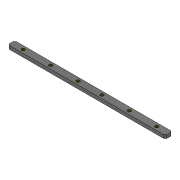
# Autodesk Inventor part: TL20240701-10100CV-003
Saved by Autodesk Inventor 2022.5 (Build 265521000, 521)
## iProperties
Category: PROFILE ASSY
Company: 현대 트랜시스
Created: 2024-04-28
Part Number: TL20240701-10100CV-003
Project: TL20240701
Checked By: 김형민
Engr Approved By: 김시현
User Status: 4 x48
Material: SS400
Description: 0
Document SubType Name: Modeling
Mfg Approved By: 호상태
Designer: 도종수
Stock Number: 003
Density: 7.85 g/cm^3
Appearance: Plating Zinc White
Folder: .\
VDS_Category: 엔지니어링
Detail Description: Processed products
Title: NUT PLATE
Subject: SW차종 시트조립라인
Author: 도종수
Revision Number: A
Autodesk Inventor part; units mm, degrees
ref_plane "YZ Plane" through (0, 0, 0) normal (1, 0, 0) x (0, 1, 0)
ref_plane "XZ Plane" through (0, 0, 0) normal (0, 1, 0) x (-1, 0, 0)
ref_plane "XY Plane" through (0, 0, 0) normal (0, 0, 1) x (1, 0, 0)
sketch "스케치52" plane through (0, 0, 0) normal (0, 0, 1) x (1, 0, 0)
  line L0 (-115, -5) -> (115, -5)
  line L1 (115, -5) -> (115, 5)
  line L2 (115, 5) -> (-115, 5)
  line L3 (-115, 5) -> (-115, -5)
  line L4 (-115, -5) -> (115, 5) construction
  line L5 (115, -5) -> (-115, 5) construction
  point P0 (0, 0)
  dimension "d480" = 230
  dimension "d481" = 10
  constraints: 12 end point, 2 midpoint, 2 parallel, 1 horizontal, 1 perpendicular
  measures "d480" distance of L1.end L2.end
  measures "d481" distance between parallel lines of L0 L2
extrude "돌출7" add sketch "스케치52" along normal mid plane 5
chamfer "모따기1" distance 2 angle 45 4 edges at (115, 5, 0) (115, -5, 0) (-115, 5, 0) (-115, -5, 0)
sketch "스케치53" plane through (0, 0, 2.5) normal (0, 0, 1) x (1, 0, 0)
  line L0 (115, -3) -> (115, 3) projected
  point P0 (0, 0)
  point P1 (-97.5, 0)
  point P2 (-57.5, 0)
  point P3 (-17.5, 0)
  point P4 (17.5, 0)
  point P5 (57.5, 0)
  point P6 (97.5, 0)
  dimension "d487" = 35
  dimension "d488" = 40
  dimension "d489" = 40
  dimension "d490" = 40
  dimension "d491" = 40
  dimension "d492" = 17.5
  constraints: 6 horizontal alignment
  measures "d487" distance of point (-17.5, 0) point (17.5, 0)
  measures "d488" distance of point (-57.5, 0) point (-17.5, 0)
  measures "d489" distance of point (-97.5, 0) point (-57.5, 0)
  measures "d490" distance of point (57.5, 0) point (17.5, 0)
  measures "d491" distance of point (97.5, 0) point (57.5, 0)
  measures "d492" distance from line of point (97.5, 0) L0
hole "구멍57" at (-97.5, 0, 2.5) at (-57.5, 0, 2.5) at (-17.5, 0, 2.5) at (17.5, 0, 2.5) at (57.5, 0, 2.5) at (97.5, 0, 2.5) direction (0, 0, -1) diameter 4.917 end through all thread size "M6x1" class "6H" standard "TS profile"
